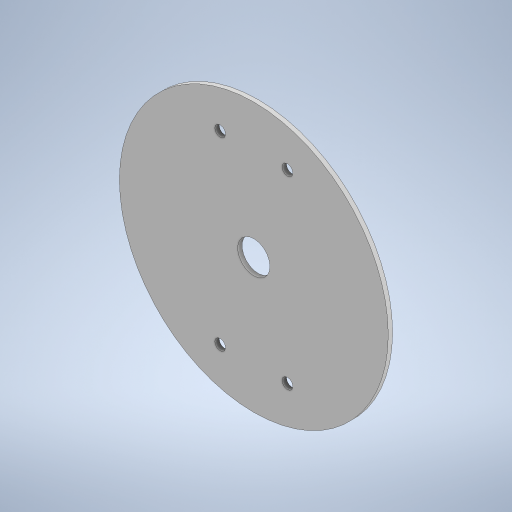
# Autodesk Inventor part: tutturgac
Saved by Autodesk Inventor 2023.2 (Build 272271000, 271)
## iProperties
Created: 2023-01-30
Part Number: tutturgac
Material: Generic
Document SubType Name: Modeling
Designer: sarp1
Density: 1 g/cm^3
Appearance: Default
Author: sarp1
Autodesk Inventor part; units mm, degrees
ref_plane "YZ Plane" through (0, 0, 0) normal (1, 0, 0) x (0, 1, 0)
ref_plane "XZ Plane" through (0, 0, 0) normal (0, 1, 0) x (-1, 0, 0)
ref_plane "XY Plane" through (0, 0, 0) normal (0, 0, 1) x (1, 0, 0)
sketch "Sketch1" plane through (0, 0, 0) normal (0, 0, 1) x (1, 0, 0)
  circle A0 centre (0, 0) radius 125
  circle A1 centre (0, 0) radius 15
  line L0 (0, 0) -> (0, 90)
  line L1 (0, 0) -> (-31.2948, 85.9819)
  line L2 (0, 0) -> (31.2948, 85.9819)
  line L3 (-125, 0) -> (125, 0) construction
  line L4 (-31.2948, 85.9819) -> (0, 90)
  line L5 (31.2948, 85.9819) -> (0, 90)
  circle A2 centre (-31.2948, 85.9819) radius 5
  circle A3 centre (31.2948, 85.9819) radius 5
  circle A4 centre (-31.2948, -85.9819) radius 5
  circle A5 centre (31.2948, -85.9819) radius 5
  dimension "d0" = 250
  dimension "d1" = 30
  dimension "d2" = 90
  dimension "d3" = 91.5
  dimension "d4" = 91.5
  dimension "d6" = 70
  dimension "d8" = 70
  dimension "d9" = 10
  dimension "d10" = 10
  constraints: 12 end point, 6 centre point, 4 coincident, 2 point on circle, 2 symmetric about line, 1 horizontal, 1 vertical, 2 other
  measures "d0" diameter of A0
  measures "d1" diameter of A1
  measures "d2" distance of L0.start L0.end
  measures "d3" distance of L0.start L1.end
  measures "d4" distance of L0.start L2.end
  measures "d6" angle of L2 L3
  measures "d8" angle of L1 L3
  measures "d9" diameter of A2
  measures "d10" diameter of A3
extrude "Extrusion1" add sketch "Sketch1" along normal blind 4 contours A0 | A1 L0 L5 A3 L2 | L1 A2 L4 L0 A1
body "Solid1"
